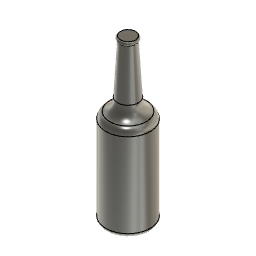
Bjórflaska v3 (Autodesk Fusion 360 design; units mm, degrees)
Autodesk Fusion 360 part; units mm, degrees
sketch "Sketch1" plane through (0, 0, 0) normal (1, 0, 0) x (0, 1, 0)
  line L0 (0, 0) -> (0, 45) construction
  line L1 (0, 0) -> (6.25, 0)
  line L2 (6.25, 0) -> (6.25, 15.1414)
  line L3 (0, 45) -> (2.1084, 45)
  line L4 (0, 45) -> (0, 0)
  arc A0 (5, 0) -> (6.25, 1.1529) centre (5.0934, 1.1529) ccw
  line L5 (2.1616, 44.0146) -> (2.9293, 30.0902)
  arc A1 (2.9293, 30.0902) -> (5.1447, 26.6121) centre (7.1308, 30.3218) ccw
  line L6 (6.25, 15.1414) -> (6.25, 24.7666)
  arc A2 (6.25, 24.7666) -> (5.1447, 26.6121) centre (4.1566, 24.7666) ccw
  circle A3 centre (2, 44.5) radius 0.5116
  dimension "d1" = 45
  dimension "d2" = 6.25
  constraint coincident L0.start L1.start
  constraint vertical L0
  constraint perpendicular L0 L1
  constraint perpendicular L0 L3
  constraint coincident L2 A0.end
  constraint coincident L1 A0.start
  constraint tangent L2 A0
  constraint tangent L5 A1
  constraint parallel L2 L6
  constraint tangent L6 A2
  constraint tangent A1 A2
  constraint coincident L3.end A3
  constraint coincident L5.start A3
  measures "d1" distance of L0.start L0.end
  measures "d2" distance of L0.start L1.end
revolve "Revolve5" add sketch "Sketch1" angle 360 about axis through (0, 0, 45) along (0, 0, -1) contours L1 L2 L3 L4 A0 L5 A1 L6 A2 A3 | L3 A3 picked at (1.8629, 44.6458)
scale "Scale1" factor 0.85 about (0, 0, 0) bodies 1
